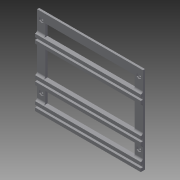
# Autodesk Inventor part: control pod wall ROUGH
Saved by Autodesk Inventor 2014 SP1 (Build 180222100, 222)
## iProperties
Created: 2017-06-22
Part Number: control pod wall ROUGH
Material: Generic
Document SubType Name: Modeling
Designer: kteo17
Density: 1 g/cm^3
Appearance: Default
Author: kteo17
Autodesk Inventor part; units mm, degrees
ref_plane "YZ Plane" through (0, 0, 0) normal (1, 0, 0) x (0, 1, 0)
ref_plane "XZ Plane" through (0, 0, 0) normal (0, 1, 0) x (-1, 0, 0)
ref_plane "XY Plane" through (0, 0, 0) normal (0, 0, 1) x (1, 0, 0)
sketch "Sketch1" plane through (0, 0, 0) normal (0, 0, 1) x (1, 0, 0)
  line L0 (0, 0) -> (161.925, 0)
  line L1 (161.925, 0) -> (161.925, 133.35)
  line L2 (161.925, 133.35) -> (0, 133.35)
  line L3 (0, 133.35) -> (0, 0)
  dimension "d0" = 161.925
  dimension "d1" = 133.35
  constraints: 8 end point, 2 parallel, 1 horizontal, 1 perpendicular
  measures "d0" distance of L2.end L1.end
  measures "d1" distance of L1.end L0.end
extrude "Extrusion1" add sketch "Sketch1" along normal blind 3.175
sketch "Sketch6" plane through (0, 0, 0) normal (0, 0, -1) x (-1, 0, 0)
  circle A0 centre (-155.575, 122.2375) radius 1.5875
  circle A1 centre (-6.35, 122.2375) radius 1.5875
  circle A2 centre (-155.575, 25.4) radius 1.5875
  circle A3 centre (-6.35, 25.4) radius 1.5875
  constraints: 4 centre point
extrude "Extrusion6" cut sketch "Sketch6" against normal blind 3.175
sketch "Sketch7" plane through (0, 0, 3.175) normal (0, 0, 1) x (1, 0, 0)
  circle A0 centre (155.575, 122.2375) radius 1.5875 projected
  circle A1 centre (6.35, 122.2375) radius 1.5875 projected
  line L0 (9.5885, 120.3678) -> (6.35, 118.498)
  line L1 (6.35, 118.498) -> (3.1115, 120.3678)
  line L2 (3.1115, 120.3678) -> (3.1115, 124.1072)
  line L3 (3.1115, 124.1072) -> (6.35, 125.977)
  line L4 (6.35, 125.977) -> (9.5885, 124.1072)
  line L5 (9.5885, 124.1072) -> (9.5885, 120.3678)
  line L6 (158.8135, 120.3678) -> (155.575, 118.498)
  line L7 (155.575, 118.498) -> (152.3365, 120.3678)
  line L8 (152.3365, 120.3678) -> (152.3365, 124.1072)
  line L9 (152.3365, 124.1072) -> (155.575, 125.977)
  line L10 (155.575, 125.977) -> (158.8135, 124.1072)
  line L11 (158.8135, 124.1072) -> (158.8135, 120.3678)
  circle A2 centre (155.575, 25.4) radius 1.5875 projected
  circle A3 centre (6.35, 25.4) radius 1.5875 projected
  line L12 (9.5885, 23.5303) -> (6.35, 21.6605)
  line L13 (6.35, 21.6605) -> (3.1115, 23.5303)
  line L14 (3.1115, 23.5303) -> (3.1115, 27.2697)
  line L15 (3.1115, 27.2697) -> (6.35, 29.1395)
  line L16 (6.35, 29.1395) -> (9.5885, 27.2697)
  line L17 (9.5885, 27.2697) -> (9.5885, 23.5303)
  line L18 (158.8135, 23.5303) -> (155.575, 21.6605)
  line L19 (155.575, 21.6605) -> (152.3365, 23.5303)
  line L20 (152.3365, 23.5303) -> (152.3365, 27.2697)
  line L21 (152.3365, 27.2697) -> (155.575, 29.1395)
  line L22 (155.575, 29.1395) -> (158.8135, 27.2697)
  line L23 (158.8135, 27.2697) -> (158.8135, 23.5303)
  point P0 (9.5885, 122.2375)
  point P1 (158.8135, 122.2375)
  constraints: 48 end point, 4 coincident, 2 midpoint, 52 other
extrude "Extrusion7" cut sketch "Sketch7" against normal blind 1.5875
sketch "Sketch11" plane through (0, 0, 3.175) normal (0, 0, 1) x (1, 0, 0)
  line L0 (161.925, 0) -> (161.925, 133.35) projected
  line L1 (0, 133.35) -> (0, 0) projected
  line L2 (0, 102.616) -> (161.925, 102.616)
  line L3 (0, 89.408) -> (161.925, 89.408)
  line L4 (0, 97.79) -> (161.925, 97.79)
  line L5 (0, 94.234) -> (161.925, 94.234)
  line L6 (0, 4.826) -> (161.925, 4.826)
  line L7 (0, 8.382) -> (161.925, 8.382)
  line L8 (0, 0) -> (161.925, 0)
  line L9 (0, 13.208) -> (161.925, 13.208)
  line L10 (0, 47.625) -> (161.925, 47.625)
  line L11 (0, 34.417) -> (161.925, 34.417)
  line L12 (0, 42.799) -> (161.925, 42.799)
  line L13 (0, 39.243) -> (161.925, 39.243)
  line L14 (161.925, 133.35) -> (0, 133.35) projected
  dimension "d83" = 4.826
  dimension "d84" = 3.556
  dimension "d85" = 4.826
  dimension "d86" = 4.826
  dimension "d87" = 3.556
  dimension "d88" = 4.826
  dimension "d89" = 4.826
  dimension "d90" = 3.556
  dimension "d91" = 4.826
  dimension "d96" = 30.861
  dimension "d98" = 35.56
  constraints: 24 end point, 7 horizontal, 1 parallel, 26 other
  measures "d83" distance between parallel lines of L6 L8
  measures "d84" distance between parallel lines of L7 L6
  measures "d85" distance between parallel lines of L9 L7
  measures "d86" distance between parallel lines of L13 L11
  measures "d87" distance between parallel lines of L12 L13
  measures "d88" distance between parallel lines of L10 L12
  measures "d89" distance between parallel lines of L5 L3
  measures "d90" distance between parallel lines of L4 L5
  measures "d91" distance between parallel lines of L2 L4
  measures "d96" distance between parallel lines of L7 L13
  measures "d98" distance between parallel lines of L4 L14
extrude "Extrusion10" add sketch "Sketch11" along normal blind 3.302 contours L8 L1 L6 L0 | L7 L1 L9 L0 | L11 L1 L13 L0 | L12 L1 L10 L0 | L3 L1 L5 L0 | L4 L1 L2 L0
sketch "Sketch15" plane through (0, 0, 3.175) normal (0, 0, 1) x (1, 0, 0)
  line L0 (0, 102.616) -> (161.925, 102.616) projected
  line L1 (12.7, 120.65) -> (149.225, 120.65)
  line L2 (149.225, 120.65) -> (149.225, 102.616)
  line L3 (149.225, 102.616) -> (12.7, 102.616)
  line L4 (12.7, 102.616) -> (12.7, 120.65)
  point P0 (0, 0)
  constraints: 8 end point, 2 parallel, 1 horizontal, 1 perpendicular, 1 point on line
sketch "Sketch16" plane through (0, 0, 3.175) normal (0, 0, 1) x (1, 0, 0)
  line L0 (0, 47.625) -> (161.925, 47.625) projected
  line L1 (161.925, 89.408) -> (0, 89.408) projected
  line L2 (12.7, 89.408) -> (149.225, 89.408)
  line L3 (149.225, 89.408) -> (149.225, 47.625)
  line L4 (149.225, 47.625) -> (12.7, 47.625)
  line L5 (12.7, 47.625) -> (12.7, 89.408)
  point P0 (0, 0)
  constraints: 8 end point, 2 parallel, 2 point on line, 1 horizontal, 1 perpendicular
sketch "Sketch17" plane through (0, 0, 3.175) normal (0, 0, 1) x (1, 0, 0)
  line L0 (0, 13.208) -> (161.925, 13.208) projected
  line L1 (161.925, 34.417) -> (0, 34.417) projected
  line L2 (12.7, 34.417) -> (149.225, 34.417)
  line L3 (149.225, 34.417) -> (149.225, 13.208)
  line L4 (149.225, 13.208) -> (12.7, 13.208)
  line L5 (12.7, 13.208) -> (12.7, 34.417)
  point P0 (0, 0)
  constraints: 8 end point, 2 parallel, 2 point on line, 1 horizontal, 1 perpendicular
extrude "Extrusion14" cut sketch "Sketch15" against normal blind 3.175
extrude "Extrusion15" cut sketch "Sketch16" against normal blind 3.175
extrude "Extrusion16" cut sketch "Sketch17" against normal blind 3.175
fillet "Fillet5" radius 3.175 10 edges at (6.35, 102.616, 3.175) (155.575, 102.616, 3.175) (155.575, 47.625, 3.175) (6.35, 47.625, 3.175) (6.35, 13.208, 3.175) (155.575, 13.208, 3.175) (6.35, 89.408, 3.175) (155.575, 89.408, 3.175) (155.575, 34.417, 3.175) (6.35, 34.417, 3.175)
body "Solid1"
